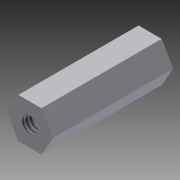
# Autodesk Inventor part: Hex Standoff 14-20 x1500
Saved by Autodesk Inventor 2013 SP2 (Build 170200200, 200)
## iProperties
Created: 2013-01-06
Part Number: Hex Standoff 14-20 x1500
Material: Aluminum 6061
Document SubType Name: Modeling
Designer: Nemo
Density: 1 g/cm^3
Author: Nemo
Autodesk Inventor part; units mm, degrees
ref_plane "YZ Plane" through (0, 0, 0) normal (1, 0, 0) x (0, 1, 0)
ref_plane "XZ Plane" through (0, 0, 0) normal (0, 1, 0) x (-1, 0, 0)
ref_plane "XY Plane" through (0, 0, 0) normal (0, 0, 1) x (1, 0, 0)
sketch "Sketch1" plane through (0, 0, 0) normal (0, 0, 1) x (1, 0, 0)
  line L0 (-3.6662, 6.35) -> (3.6662, 6.35)
  line L1 (3.6662, 6.35) -> (7.3323, 0)
  line L2 (7.3323, 0) -> (3.6662, -6.35)
  line L3 (3.6662, -6.35) -> (-3.6662, -6.35)
  line L4 (-3.6662, -6.35) -> (-7.3323, 0)
  line L5 (-7.3323, 0) -> (-3.6662, 6.35)
  point P0 (0, 0)
  point P1 (0, 0)
  dimension "d0" = 12.7
  constraints: 12 end point, 1 coincident, 1 horizontal, 13 other
  measures "d0" distance between parallel lines of L0 L3
extrude "Extrusion1" add sketch "Sketch1" along normal mid plane 38.1
sketch "Sketch2" plane through (0, 0, 19.05) normal (0, 0, 1) x (1, 0, 0)
  point P0 (0, 0)
  point P1 (0, 0)
  constraints: 1 coincident
hole "Hole1" at (0, 0, 19.05) direction (0, 0, -1) diameter 4.9784 end through all thread size "1/4-20 UNC" class "2B" standard "ANSI Unified Screw Threads"
body "Solid1"
